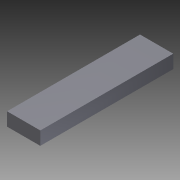
# Autodesk Inventor part: 2431
Saved by Autodesk Inventor 2011 SP1 (Build 150282100, 282)
## iProperties
Company: Allseas Engineering BV
Created: 2011-09-26
Part Number: 2431
Cost Center: 0 kg
Material: Steel
Document SubType Name: Modeling
Designer: PMe
Authority: 0 mm^3
Stock Number: =<Filenr>_<Document number>
Density: 7.85 g/cm^3
Act. Code: DW000
SaveDate: 2011-07-28
SaveTime: 18:32
FileName: Standard
TotalMass: 0 kg
TotalVolume: 0 mm^3
Subject: =<Title><TITLE 1_2> <TITLE 2_2>
Author: PMe
Autodesk Inventor part; units mm, degrees
ref_plane "YZ Plane" through (0, 0, 0) normal (1, 0, 0) x (0, 1, 0)
ref_plane "XZ Plane" through (0, 0, 0) normal (0, 1, 0) x (-1, 0, 0)
ref_plane "XY Plane" through (0, 0, 0) normal (0, 0, 1) x (1, 0, 0)
sketch "Sketch1" plane through (0, 0, 0) normal (0, 0, 1) x (1, 0, 0)
  line L0 (-4, 16) -> (4, 16)
  line L1 (4, 16) -> (4, -16)
  line L2 (4, -16) -> (-4, -16)
  line L3 (-4, -16) -> (-4, 16)
  point P0 (0, 0)
  dimension "d0" = 8
  dimension "d1" = 32
  dimension "d2" = 4
  dimension "d3" = 16
  constraints: 8 end point, 2 parallel, 1 horizontal, 1 perpendicular
  measures "d0" distance of L1.end L2.end
  measures "d1" distance of L0.end L1.end
  measures "d2" distance from line of point (0, 0) L1
  measures "d3" distance from line of point (0, 0) L2
extrude "Extrusion1" add sketch "Sketch1" along normal blind 3.2
shell "Shell1" thickness 1.5 removed faces 1 at (1.3333, 5.3333, 0)
sketch "Sketch2" plane through (0, 0, 3.2) normal (0, 0, 1) x (1, 0, 0)
  circle A0 centre (0, -12) radius 2.5
  line L0 (4, 16) -> (4, -16) projected
  line L1 (4, -16) -> (-4, -16) projected
  dimension "d7" = 5
  dimension "d10" = 4
  dimension "d11" = 4
  constraints: 1 centre point, 1 coincident
  measures "d7" diameter of A0
  measures "d10" distance from line of L1 point (0, -12)
  measures "d11" distance from line of L0 point (0, -12)
extrude "Extrusion2" [suppressed]
sketch "Sketch3" plane through (2.5, -14.5, 1.7) normal (0, 0, -1) x (-1, 0, 0)
  circle A0 centre (2.5, 2.5) radius 1.2
  point P0 (2.5, 14.5)
  dimension "d18" = 2.4
  constraints: 1 centre point
  measures "d18" diameter of A0
extrude "Extrusion3" [suppressed]
pattern_linear "Rectangular Pattern1" [suppressed]
sketch "Sketch4" plane through (2.5, -14.5, 1.7) normal (0, 0, -1) x (-1, 0, 0)
  line L0 (0, 29) -> (0, 0) projected
  line L1 (0, 0) -> (5, 0) projected
  circle A0 centre (6.5, 6.5) radius 3.15
  circle A1 centre (6.5, 6.5) radius 2.5
  point P0 (2.5, 14.5)
  dimension "d21" = 6.5
  dimension "d22" = 6.5
  dimension "d25" = 5
  dimension "d26" = 6.3
  constraints: 2 centre point, 1 coincident
  measures "d21" distance from line of L1 A0.centre
  measures "d22" distance from line of L0 A0.centre
  measures "d25" diameter of A1
  measures "d26" diameter of A0
extrude "Extrusion4" [suppressed]
pattern_linear "Rectangular Pattern2" [suppressed]
equation "\"d0\" = 8 * WIDTH"
equation "\"d1\" = 8 * LENGTH"
equation "\"d2\" = 0.5 * d0"
equation "\"d3\" = 0.5 * d1"
equation "\"d4\" = HEIGHT"
equation "\"d21\" = 0.5 * d23 + 0.5 * d24"
equation "\"d22\" = d21"
equation "\"WIDTH\" = 1"
equation "\"HEIGHT\" = 3.2"
equation "\"LENGTH\" = 4"
equation "\"d23\" = 10.5"
equation "\"d24\" = 2.5"
body "Solid1"
